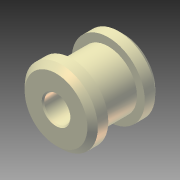
# Autodesk Inventor part: D-030
Saved by Autodesk Inventor 2015 (Build 190159000, 159)
## iProperties
Company: MARCHA TECHNOLOGY
Created: 2013-10-24
Part Number: D-030
Document SubType Name: Modeling
Designer: O.Martin
Density: 1 g/cm^3
Mass: 1.32988 g
Surface Area: 10.7893 cm^2
Volume: 1.32988 cm^3
Project: WITBOXprinter_K01
Description: RODILLO CORREA X
Stock Number: 28655
Material: Generic
Appearance: Nylon 6
Author: O.Martin
Autodesk Inventor part; units mm, degrees
ref_plane "YZ Plane" through (0, 0, 0) normal (1, 0, 0) x (0, 1, 0)
ref_plane "XZ Plane" through (0, 0, 0) normal (0, 1, 0) x (-1, 0, 0)
ref_plane "XY Plane" through (0, 0, 0) normal (0, 0, 1) x (1, 0, 0)
sketch "Boceto1" plane through (0, 0, 0) normal (0, 0, 1) x (1, 0, 0)
  line L0 (0, 6.5) -> (7, 6.5)
  line L1 (7, 6.5) -> (7, -6.5)
  line L2 (7, -6.5) -> (0, -6.5)
  line L3 (0, -6.5) -> (0, 6.5)
  line L4 (7, 3.5) -> (5.5, 3.5)
  line L5 (5.5, 3.5) -> (5.5, -3.5)
  line L6 (5.5, -3.5) -> (7, -3.5)
  line L7 (7, -3.5) -> (7, 3.5)
  line L8 (2.5, 6.5) -> (2.5, -6.5)
  point P0 (0, 0)
  point P1 (7, 0)
  point P2 (0, 0)
  dimension "d0" = 7
  dimension "d1" = 13
  dimension "d2" = 14
  dimension "d3" = 11
  dimension "d5" = 5
  constraints: 18 end point, 4 parallel, 3 midpoint, 3 perpendicular, 3 point on line, 2 horizontal, 1 coincident
  measures "d0" distance of L4.end L5.end
  measures "d1" distance of L0.end L1.end
  measures "d2" diameter of L1 L3
  measures "d3" diameter of L5 L3
  measures "d5" diameter of L8 L3
revolve "Revolución1" add sketch "Boceto1" angle 360 about axis through (0, -6.5, 0) along (0, 1, 0) contours L0 L1 L4 L5 L6 L2 L8
chamfer "Chaflán1" distance 0.25 angle 45 2 edges at (-2.5, -6.5, 0) (-2.5, 6.5, 0)
chamfer "Chaflán2" distance 1 angle 45 2 edges at (-7, -6.5, 0) (-7, 6.5, 0)
body "Solid1"
